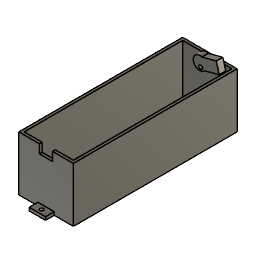
BATT_LOCK_ASSY (Autodesk Fusion 360 design; units mm, degrees)
Autodesk Fusion 360 part; units mm, degrees
sketch "Sketch1" plane through (0, 0, 0) normal (0, 0, 1) x (1, 0, 0) in component "BATT_LOCK_TRAY_V1"
  line L0 (-25, -75) -> (25, -75)
  line L1 (25, -75) -> (25, 75)
  line L2 (25, 75) -> (-25, 75)
  line L3 (-25, 75) -> (-25, -75)
  line L4 (-22.5, -72.5) -> (22.5, -72.5)
  line L5 (22.5, -72.5) -> (22.5, 72.5)
  line L6 (22.5, 72.5) -> (-22.5, 72.5)
  line L7 (-22.5, 72.5) -> (-22.5, -72.5)
extrude "Extrude1" add sketch "Sketch1" along normal blind 3 contours L0 L1 L2 L3 | L4 L5 L6 L7 makes body 1 in component "BATT_LOCK_TRAY_V1"
extrude "Extrude2" add sketch "Sketch1" along normal blind 50 bodies 1 in component "BATT_LOCK_TRAY_V1"
sketch "Sketch2" plane through (0, 0, 0) normal (0, 0, 1) x (1, 0, 0) in component "BATT_LOCK_TRAY_V1"
  line L0 (-7.5, 75) -> (7.5, 75)
  line L1 (7.5, 75) -> (7.5, 83)
  line L2 (7.5, 83) -> (-7.5, 83)
  line L3 (-7.5, 83) -> (-7.5, 75)
  line L4 (-7.5, -83) -> (7.5, -83)
  line L5 (7.5, -83) -> (7.5, -75)
  line L6 (7.5, -75) -> (-7.5, -75)
  line L7 (-7.5, -75) -> (-7.5, -83)
extrude "Extrude3" add sketch "Sketch2" along normal blind 3 bodies 1 in component "BATT_LOCK_TRAY_V1"
sketch "Sketch3" plane through (0, 0, 0) normal (0, 0, 1) x (1, 0, 0) in component "BATT_LOCK_TRAY_V1"
  circle A0 centre (0, 79) radius 1.7
  circle A1 centre (0, -79) radius 1.7
extrude "Extrude4" cut sketch "Sketch3" along normal blind 5 bodies 1 in component "BATT_LOCK_TRAY_V1"
ref_plane "WorkPlane1" through (0, 73.75, 0) normal (0, 1, 0) x (0, 0, 1) in component "BATT_LOCK_TRAY_V1"
sketch "Sketch4" plane through (0, 73.75, 0) normal (0, 1, 0) x (1, 0, 0) in component "BATT_LOCK_TRAY_V1"
  circle A0 centre (0, -43) radius 1.7
extrude "Extrude5" cut sketch "Sketch4" along normal mid plane 12 bodies 1 in component "BATT_LOCK_TRAY_V1"
ref_plane "WorkPlane2" through (0, -73.75, 0) normal (0, 1, 0) x (0, 0, 1) in component "BATT_LOCK_TRAY_V1"
sketch "Sketch5" plane through (0, -73.75, 0) normal (0, 1, 0) x (1, 0, 0) in component "BATT_LOCK_TRAY_V1"
  line L0 (-6, -42) -> (6, -42)
  line L1 (6, -42) -> (6, -50)
  line L2 (6, -50) -> (-6, -50)
  line L3 (-6, -50) -> (-6, -42)
extrude "Extrude6" cut sketch "Sketch5" along normal mid plane 12 bodies 1 in component "BATT_LOCK_TRAY_V1"
sketch "Sketch6" plane through (0, 0, 0) normal (0, 0, 1) x (1, 0, 0) in component "BATT_LOCK_TRAY_V1"
  line L0 (-2, -69) -> (2, -69)
  line L1 (2, -69) -> (2, -57)
  line L2 (2, -57) -> (-2, -57)
  line L3 (-2, -57) -> (-2, -69)
extrude "Extrude7" cut sketch "Sketch6" along normal blind 4 bodies 1 in component "BATT_LOCK_TRAY_V1"
sketch "Sketch1 (2)" plane through (0, 0, 0) normal (0, 0, 1) x (1, 0, 0) in component "BATT_LOCK_CAM_V2"
  line L0 (0, -5) -> (17, -5)
  line L1 (17, -5) -> (17, 5)
  line L2 (17, 5) -> (0, 5)
  line L3 (0, 5) -> (0, -5)
  circle A0 centre (0, 0) radius 6
extrude "Extrude1'" add sketch "Sketch1 (2)" along normal blind 6 separate body makes body 2 in component "BATT_LOCK_CAM_V2"
sketch "Sketch2 (2)" plane through (0, 0, 0) normal (0, 0, 1) x (1, 0, 0) in component "BATT_LOCK_CAM_V2"
  circle A0 centre (0, 3) radius 1.7
extrude "Extrude8" cut sketch "Sketch2 (2)" along normal blind 8 bodies 1 in component "BATT_LOCK_TRAY_V1"
extrude "Extrude2'" cut sketch "Sketch2 (2)" along normal blind 8 bodies 2 in component "BATT_LOCK_CAM_V2"
component "BATT_LOCK_TRAY_V1" placed x (1, 0, 0) y (0, 1, 0) z (0, 0, 1) at (0, 0, 0)
component "BATT_LOCK_CAM_V2" placed x (0.965926, 0, 0.258819) y (0.258819, 0, -0.965926) z (0, 1, 0) at (-0.7765, 66.5, 45.8978)
